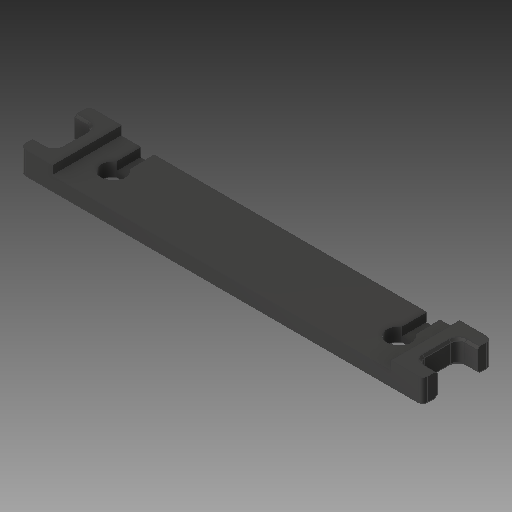
# Autodesk Inventor part: LR Spigot Plate
Saved by Autodesk Inventor 2019 (Build 230136000, 136)
## iProperties
Created: 2016-01-25
Part Number: LR Spigot Plate
Material: Acetal Resin, Black
Document SubType Name: Modeling
Designer: IEUser
Density: 1.425 g/cm^3
Appearance: Smooth - Black
Author: IEUser
Autodesk Inventor part; units mm, degrees
ref_plane "YZ Plane" through (0, 0, 0) normal (1, 0, 0) x (0, 1, 0)
ref_plane "XZ Plane" through (0, 0, 0) normal (0, 1, 0) x (-1, 0, 0)
ref_plane "XY Plane" through (0, 0, 0) normal (0, 0, 1) x (1, 0, 0)
sketch "Body Outline" plane through (0, 0, 0) normal (0, 1, 0) x (-1, 0, 0)
  line L0 (88, -15) -> (-88, -15)
  line L1 (-88, -15) -> (-88, 15)
  line L2 (-88, 15) -> (88, 15)
  line L3 (88, 15) -> (88, -15)
  point P0 (0, 0)
  dimension "d0" = 30
  dimension "d1" = 15
  dimension "d2" = 176
  dimension "d3" = 88
  constraints: 8 end point, 2 parallel, 1 horizontal, 1 perpendicular
  measures "d0" distance of L2.end L0.start
  measures "d1" distance from line of point (0, 0) L0
  measures "d2" distance of L0.start L0.end
  measures "d3" distance from line of point (0, 0) L3
extrude "Body" add sketch "Body Outline" along normal blind 10
sketch "Body Cutout Outline" plane through (0, 10, 0) normal (0, 1, 0) x (1, 0, 0)
  line L0 (-74, 15) -> (74, 15)
  line L1 (74, 15) -> (74, -15)
  line L2 (74, -15) -> (-74, -15)
  line L3 (-74, -15) -> (-74, 15)
  line L4 (-88, 15) -> (-88, -15) projected
  line L5 (88, -15) -> (88, 15) projected
  line L6 (88, 15) -> (-88, 15) projected
  line L7 (-88, -15) -> (88, -15) projected
  point P0 (0, 0)
  dimension "d6" = 14
  dimension "d7" = 14
  dimension "d8" = 0
  dimension "d9" = 0
  constraints: 8 end point, 2 parallel, 1 horizontal, 1 perpendicular
  measures "d6" distance between parallel lines of L4 L3
  measures "d7" distance between parallel lines of L5 L1
  measures "d8" distance between parallel lines of L6 L0
  measures "d9" distance between parallel lines of L7 L2
extrude "Body Cutout" cut sketch "Body Cutout Outline" against normal blind 4 contours L0 L1 L2 L3
sketch "Rail Cutouts Outline" plane through (0, 0, 0) normal (0, -1, 0) x (1, 0, 0)
  line L0 (99.5, -8.75) -> (79.5, -8.75)
  line L1 (79.5, -8.75) -> (79.5, 8.75)
  line L2 (79.5, 8.75) -> (99.5, 8.75)
  line L3 (99.5, 8.75) -> (99.5, -8.75)
  line L4 (88, -15) -> (88, 15) projected
  line L5 (-99.5, -8.75) -> (-79.5, -8.75)
  line L6 (-79.5, -8.75) -> (-79.5, 8.75)
  line L7 (-79.5, 8.75) -> (-99.5, 8.75)
  line L8 (-99.5, 8.75) -> (-99.5, -8.75)
  line L9 (-88, 15) -> (-88, -15) projected
  point P0 (0, 0)
  dimension "d12" = 8.5
  dimension "d13" = 17.5
  dimension "d14" = 8.75
  dimension "d16" = 8.5
  dimension "d17" = 20
  dimension "d18" = 20
  dimension "d19" = 17.5
  dimension "d20" = 8.75
  constraints: 16 end point, 4 parallel, 2 horizontal, 2 perpendicular
  measures "d12" distance between parallel lines of L4 L1
  measures "d13" distance of L2.end L0.start
  measures "d14" distance from line of point (0, 0) L0
  measures "d16" distance between parallel lines of L9 L6
  measures "d17" distance of L0.start L0.end
  measures "d18" distance of L5.start L5.end
  measures "d19" distance of L7.end L5.start
  measures "d20" distance from line of point (0, 0) L5
extrude "Rail Cutouts" cut sketch "Rail Cutouts Outline" along normal through all both and the other way through all
sketch "Spigot Cutouts Outline" plane through (0, 6, 0) normal (0, 1, 0) x (1, 0, 0)
  arc A0 (-65.5, 4.3084) -> (-59.5, 4.3084) centre (-62.5, 0) ccw
  line L0 (-65.5, 15) -> (-59.5, 15)
  line L1 (-59.5, 15) -> (-59.5, 4.3084)
  line L2 (-65.5, 4.3084) -> (-65.5, 15)
  line L3 (-74, 15) -> (74, 15) projected
  arc A1 (59.5, 4.3084) -> (65.5, 4.3084) centre (62.5, 0) ccw
  line L4 (59.5, 15) -> (65.5, 15)
  line L5 (65.5, 15) -> (65.5, 4.3084)
  line L6 (59.5, 4.3084) -> (59.5, 15)
  point P0 (0, 0)
  dimension "d23" = 6
  dimension "d24" = 62.5
  dimension "d25" = 0
  dimension "d26" = 0
  dimension "d27" = 5.25
  dimension "d28" = 3
  dimension "d29" = 6
  dimension "d30" = 3
  dimension "d31" = 5.25
  dimension "d32" = 0
  dimension "d33" = 0
  dimension "d34" = 62.5
  constraints: 12 end point, 4 point on circle, 2 centre point, 2 horizontal, 2 parallel, 2 perpendicular
  measures "d23" distance of L0.start L0.end
  measures "d24" distance of point (0, 0) A0.centre
  measures "d25" distance between parallel lines of L0 L3
  measures "d26" vertical distance of A0.centre point (0, 0)
  measures "d27" radius of A0
  measures "d28" distance from line of A0.centre L2
  measures "d29" distance of L4.start L4.end
  measures "d30" distance from line of L5 A1.centre
  measures "d31" radius of A1
  measures "d32" vertical distance of point (0, 0) A1.centre
  measures "d33" distance between parallel lines of L3 L4
  measures "d34" distance of A1.centre point (0, 0)
extrude "Spigot Cutouts" cut sketch "Spigot Cutouts Outline" along normal through all both and the other way through all
sketch "Spigot Supports Outline" plane through (0, 0, 0) normal (0, -1, 0) x (1, 0, 0)
  line L0 (-65.5, -4.3084) -> (-59.5, -4.3084)
  line L1 (-59.5, -4.3084) -> (-59.5, -15)
  line L2 (-59.5, -15) -> (-65.5, -15)
  line L3 (-65.5, -15) -> (-65.5, -4.3084)
  line L4 (-65.5, -15) -> (-65.5, -4.3084) projected
  line L5 (-59.5, -4.3084) -> (-59.5, -15) projected
  line L6 (-88, -15) -> (-65.5, -15) projected
  line L7 (59.5, -4.3084) -> (65.5, -4.3084)
  line L8 (65.5, -4.3084) -> (65.5, -15)
  line L9 (65.5, -15) -> (59.5, -15)
  line L10 (59.5, -15) -> (59.5, -4.3084)
  line L11 (65.5, -4.3084) -> (65.5, -15) projected
  line L12 (59.5, -15) -> (59.5, -4.3084) projected
  line L13 (-59.5, -15) -> (59.5, -15) projected
  point P0 (0, 0)
  dimension "d37" = 0
  dimension "d38" = 0
  dimension "d39" = 0
  dimension "d40" = 0
  dimension "d41" = 0
  dimension "d42" = 0
  dimension "d43" = 0
  dimension "d44" = 0
  constraints: 16 end point, 4 parallel, 2 horizontal, 2 perpendicular
  measures "d37" distance between parallel lines of L4 L3
  measures "d38" distance from line of L0 L4.end
  measures "d39" distance between parallel lines of L5 L1
  measures "d40" distance between parallel lines of L6 L2
  measures "d41" distance between parallel lines of L11 L8
  measures "d42" distance from line of L11.start L7
  measures "d43" distance between parallel lines of L10 L12
  measures "d44" distance between parallel lines of L13 L9
extrude "Spigot Supports" add sketch "Spigot Supports Outline" against normal blind 2
fillet "Body Fillet" radius 3 4 edges at (-79.5, 5, -8.75) (-79.5, 5, 8.75) (79.5, 5, -8.75) (79.5, 5, 8.75)
fillet "Body Fillet" radius 2 4 edges at (-88, 5, 15) (-88, 5, -15) (88, 5, -15) (88, 5, 15)
chamfer "Rail Cutouts Chamfer" distance 1 angle 45 20 edges at (-85.25, 10, -8.75) (-80.3787, 10, -7.8713) (-79.5, 10, 0) (-80.3787, 10, 7.8713) (-85.25, 10, 8.75) (-85.25, 0, -8.75) (-80.3787, 0, -7.8713) (-79.5, 0, 0) (-80.3787, 0, 7.8713) (-85.25, 0, 8.75) (85.25, 10, -8.75) (80.3787, 10, -7.8713) (79.5, 10, 0) (80.3787, 10, 7.8713) (85.25, 10, 8.75) (85.25, 0, 8.75) (80.3787, 0, 7.8713) (79.5, 0, 0) (80.3787, 0, -7.8713) (85.25, 0, -8.75)
equation "\"d1\" = 0.5 * d0"
equation "\"d3\" = 0.5 * d2"
equation "\"d7\" = d6"
equation "\"d14\" = 0.5 * d13"
equation "\"d16\" = d12"
equation "\"d18\" = d17"
equation "\"d19\" = d13"
equation "\"d20\" = 0.5 * d19"
equation "\"d28\" = 0.5 * d23"
equation "\"d29\" = d23"
equation "\"d30\" = d28"
equation "\"d31\" = d27"
equation "\"d34\" = d24"
body "Solid1"
